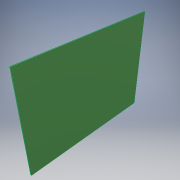
# Autodesk Inventor part: PCB#01
Saved by Autodesk Inventor 2018 (Build 220112000, 112)
## iProperties
Created: 2025-02-15
Part Number: PCB#01
Material: LCP plast
Document SubType Name: Modeling
Designer: Jozko Mrkvicka
Density: 1.626 g/cm^3
Appearance: Hladká – bílá
Author: Jozko Mrkvicka
Autodesk Inventor part; units mm, degrees
ref_plane "YZ Plane" through (0, 0, 0) normal (1, 0, 0) x (0, 1, 0)
ref_plane "XZ Plane" through (0, 0, 0) normal (0, 1, 0) x (-1, 0, 0)
ref_plane "XY Plane" through (0, 0, 0) normal (0, 0, 1) x (1, 0, 0)
sketch "Náčrt1" plane through (0, 0, 0) normal (1, 0, 0) x (0, 1, 0)
  line L0 (0, 0) -> (228.6, 0)
  line L1 (228.6, 0) -> (228.6, -304.8)
  line L2 (228.6, -304.8) -> (0, -304.8)
  line L3 (0, -304.8) -> (0, 0)
  dimension "d0" = 228.6
  dimension "d1" = 304.8
  constraints: 8 end point, 2 parallel, 1 horizontal, 1 perpendicular
  measures "d0" distance of L1.end L2.end
  measures "d1" distance of L2.end L0.start
extrude "Vysunutí1" add sketch "Náčrt1" along normal blind 2.54
equation "\"d0\" = width"
equation "\"d1\" = length"
equation "\"d2\" = gPcbThickness"
equation "\"length\" = 304.8"
equation "\"width\" = 228.6"
equation "\"gPcbThickness\" = 2.54"
